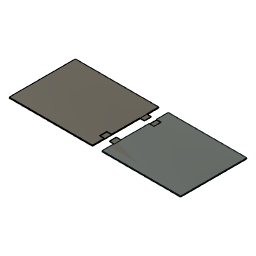
_Bottom Slide.52f3d79a-d360-466b-9179-13a9d49c522c (Autodesk Fusion 360 design; units mm, degrees)
Autodesk Fusion 360 part; units mm, degrees
sketch "Sketch1" plane through (0, 0, 0) normal (0, 0, 1) x (1, 0, 0)
  line L0 (0, 0) -> (340, 0)
  line L1 (340, 0) -> (340, 139)
  line L2 (340, 139) -> (0, 139)
  line L3 (0, 139) -> (0, 0)
  dimension "d1" = 340
  dimension "d2" = 139
  constraint horizontal L0
  constraint vertical L1
  constraint horizontal L2
  constraint vertical L3
  constraint coincident L0.start L3.end
  measures "d1" distance of L0.start L0.end
  measures "d2" distance of L0.start L2.end
extrude "Extrude1" add sketch "Sketch1" along normal blind 1.9 makes body 1
sketch "Sketch2" plane through (0, 0, 1.9) normal (0, 0, 1) x (-1, 0, 0)
  line L0 (0, -139) -> (0, 0)
  line L1 (0, 0) -> (-340, 0)
  line L2 (-340, 0) -> (-340, -139)
  line L3 (-340, -139) -> (0, -139)
  line L4 (-175, 0) -> (-175, -139)
  dimension "d5" = 175
  constraint coincident L1 L4.start
  constraint coincident L3 L4.end
  constraint perpendicular L3 L4
  measures "d5" distance of L0.start L4.end
split "Split1" by curves path "Sketch2" along L4 bodies 1 makes body 2 at (230, 92.6667, 0)
move_body "Move1" bodies 2 to x (1, 0, 0) y (0, 1, 0) z (0, 0, 1) at (20, 0, 0)
sketch "Sketch3" plane through (0, 0, 1.9) normal (0, 0, 1) x (-1, 0, 0)
  line L0 (-175, 0) -> (-175, -139)
  line L1 (-175, -139) -> (0, -139)
  line L2 (0, -139) -> (0, 0)
  line L3 (0, 0) -> (-175, 0)
  line L4 (-175, -25) -> (-165, -25)
  line L5 (-165, -25) -> (-165, -40)
  line L6 (-165, -40) -> (-175, -40)
  dimension "d6" = 10
  dimension "d7" = 15
  dimension "d8" = 25
  constraint coincident L0 L4.start
  constraint perpendicular L0 L4
  constraint perpendicular L4 L5
  constraint coincident L0 L6.end
  constraint perpendicular L0 L6
  measures "d6" distance of L4.start L4.end
  measures "d7" distance of L4.end L5.end
  measures "d8" distance of L3 L4
extrude "Extrude2" cut sketch "Sketch3" against normal blind 1 contours L0 L4 L5 L6 bodies 1
sketch "Sketch4" plane through (0, 0, 1.9) normal (0, 0, 1) x (-1, 0, 0)
  line L0 (-195, -139) -> (-195, 0)
  line L1 (-195, 0) -> (-360, 0)
  line L2 (-360, 0) -> (-360, -139)
  line L3 (-360, -139) -> (-195, -139)
  line L4 (-195, -114) -> (-205, -114)
  line L5 (-205, -114) -> (-205, -99)
  line L6 (-205, -99) -> (-195, -99)
  line L7 (-195, -99) -> (-195, -114)
  dimension "d11" = 15
  dimension "d12" = 25
  dimension "d13" = 10
  constraint horizontal L4
  constraint vertical L5
  constraint horizontal L6
  constraint vertical L7
  constraint coincident L0 L4.start
  measures "d11" distance of L4.end L5.end
  measures "d12" distance of L3 L4
  measures "d13" distance of L5.end L6.end
extrude "Extrude3" cut sketch "Sketch4" against normal blind 1 contours L0 L4 L5 L6 L7 bodies 2
sketch "Sketch5" plane through (0, 0, 1.9) normal (0, 0, 1) x (-1, 0, 0)
  line L0 (-205, -99) -> (-195, -99)
  line L1 (-195, -99) -> (-195, 0)
  line L2 (-195, 0) -> (-360, 0)
  line L3 (-360, 0) -> (-360, -139)
  line L4 (-360, -139) -> (-195, -139)
  line L5 (-195, -139) -> (-195, -114)
  line L6 (-195, -114) -> (-205, -114)
  line L7 (-205, -114) -> (-205, -99)
sketch "Sketch6" plane through (0, 0, 1.9) normal (0, 0, 1) x (-1, 0, 0)
sketch "Sketch7" plane through (195, 0, 0) normal (-1, 0, 0) x (0, -1, 0)
  line L0 (-99, 1.9) -> (-99, 0.9)
  line L1 (-99, 0.9) -> (-114, 0.9)
  line L2 (-114, 0.9) -> (-114, 1.9)
  line L3 (-114, 1.9) -> (-139, 1.9)
  line L4 (-139, 1.9) -> (-139, 0)
  line L5 (-139, 0) -> (0, 0)
  line L6 (0, 0) -> (0, 1.9)
  line L7 (0, 1.9) -> (-99, 1.9)
  line L8 (-39.8, 1.9) -> (-25.2, 1.9)
  line L9 (-25.2, 1.9) -> (-25.2, 1.1)
  line L10 (-25.2, 1.1) -> (-39.8, 1.1)
  line L11 (-39.8, 1.1) -> (-39.8, 1.9)
  dimension "d16" = 0.8
  dimension "d17" = 14.6
  dimension "d18" = 25.2
  constraint horizontal L8
  constraint vertical L9
  constraint horizontal L10
  constraint vertical L11
  constraint coincident L7 L8.start
  measures "d16" distance of L8.start L10.end
  measures "d17" distance of L8.start L8.end
  measures "d18" distance of L6 L8.end
extrude "Extrude4" add sketch "Sketch7" along normal blind 9.8 contours L7 L8 L9 L10 L11 bodies 2
sketch "Sketch8" plane through (175, 0, 0) normal (1, 0, 0) x (0, 1, 0)
  line L0 (25, 0.9) -> (25, 1.9)
  line L1 (25, 1.9) -> (0, 1.9)
  line L2 (0, 1.9) -> (0, 0)
  line L3 (0, 0) -> (139, 0)
  line L4 (139, 0) -> (139, 1.9)
  line L5 (139, 1.9) -> (40, 1.9)
  line L6 (40, 1.9) -> (40, 0.9)
  line L7 (40, 0.9) -> (25, 0.9)
  line L8 (99.2, 1.9) -> (113.8, 1.9)
  line L9 (113.8, 1.9) -> (113.8, 1.1)
  line L10 (113.8, 1.1) -> (99.2, 1.1)
  line L11 (99.2, 1.1) -> (99.2, 1.9)
  dimension "d21" = 14.6
  dimension "d22" = 25.2
  dimension "d23" = 0.8
  constraint horizontal L8
  constraint vertical L9
  constraint horizontal L10
  constraint vertical L11
  constraint coincident L5 L8.start
  measures "d21" distance of L8.start L8.end
  measures "d22" distance of L4 L9
  measures "d23" distance of L8.end L9.end
extrude "Extrude5" add sketch "Sketch8" along normal blind 9.8 contours L5 L8 L9 L10 L11 bodies 1
copy_body "Body->Comp1" bodies 1 removing the originals makes body 3 in component "Component"
copy_body "Body->Comp2" bodies 2 removing the originals makes body 4 in component "Component'"
component "Component" placed x (1, 0, 0) y (0, 1, 0) z (0, 0, 1) at (0, 0, 0)
component "Component'" placed x (1, 0, 0) y (0, 1, 0) z (0, 0, 1) at (0, 0, 0)
